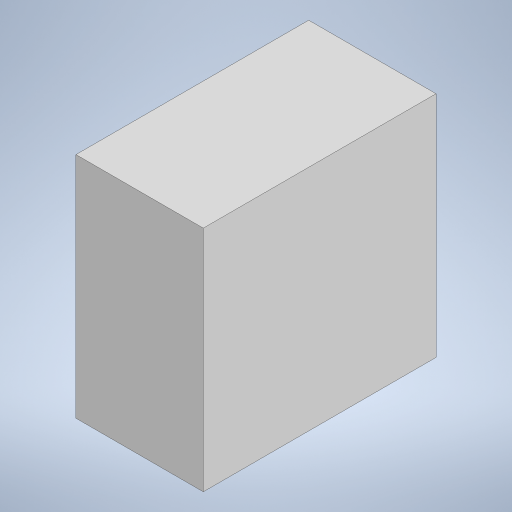
# Autodesk Inventor part: servoHolderBase
Saved by Autodesk Inventor 2024 (Build 280153000, 153)
## iProperties
Created: 2024-08-21
Part Number: servoHolderBase
Material: Generic
Document SubType Name: Modeling
Designer: omiye
Density: 1 g/cm^3
Appearance: Default
Author: omiye
Autodesk Inventor part; units mm, degrees
ref_plane "YZ Plane" through (0, 0, 0) normal (1, 0, 0) x (0, 1, 0)
ref_plane "XZ Plane" through (0, 0, 0) normal (0, 1, 0) x (-1, 0, 0)
ref_plane "XY Plane" through (0, 0, 0) normal (0, 0, 1) x (1, 0, 0)
sketch "Sketch1" plane through (0, 0, 0) normal (1, 0, 0) x (0, 1, 0)
  line L0 (-12, 12.25) -> (12, 12.25)
  line L1 (12, 12.25) -> (12, -12.25)
  line L2 (12, -12.25) -> (-12, -12.25)
  line L3 (-12, -12.25) -> (-12, 12.25)
  line L4 (-12, 12.25) -> (12, -12.25) construction
  line L5 (12, 12.25) -> (-12, -12.25) construction
  line L6 (-13, -13.25) -> (13, -13.25)
  line L7 (13, -13.25) -> (13, 13.25)
  line L8 (13, 13.25) -> (-13, 13.25)
  line L9 (-13, 13.25) -> (-13, -13.25)
  line L10 (-13, -13.25) -> (13, 13.25) construction
  line L11 (13, -13.25) -> (-13, 13.25) construction
  point P0 (0, 0)
  dimension "d0" = 24
  dimension "d1" = 24.5
  dimension "d2" = 26
  dimension "d3" = 26.5
  constraints: 24 end point, 4 midpoint, 4 parallel, 2 horizontal, 2 perpendicular
  measures "d0" distance of L1.end L2.end
  measures "d1" distance of L0.end L1.end
  measures "d2" distance of L8.end L7.end
  measures "d3" distance of L7.end L6.end
extrude "Extrusion1" add sketch "Sketch1" along normal blind 14.5
sketch "Sketch2" plane through (0, 13, 13.25) normal (0, 1, 0) x (1, 0, 0)
  line L0 (0, 26.5) -> (14.5, 26.5) projected
  line L1 (0, 0) -> (14.5, 0) projected
  line L2 (14.5, 26.5) -> (12.5, 26.5)
  line L3 (12.5, 26.5) -> (12.5, 0)
  line L4 (12.5, 0) -> (14.5, 0)
  line L5 (14.5, 0) -> (14.5, 26.5)
  point P0 (0, 13.25)
  dimension "d6" = 2
  constraints: 8 end point, 2 parallel, 1 horizontal, 1 perpendicular, 1 point on line
  measures "d6" distance of L4.end L3.end
extrude "Extrusion2" add sketch "Sketch2" against normal blind 26
sketch "Sketch3" plane through (0, 0, 0) normal (-1, 0, 0) x (0, 0, 1)
  point P0 (0, 0)
body "Solid1"
